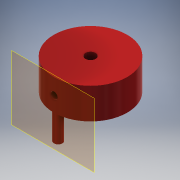
# Autodesk Inventor part: Cup_Dispenser_Transmission
Saved by Autodesk Inventor 2016 (Build 200138000, 138)
## iProperties
Created: 2015-07-09
Part Number: Cup_Dispenser_Transmission
Material: Generic
Document SubType Name: Modeling
Designer: 3DPrinterUser
Density: 1 g/cm^3
Appearance: Light Red
Author: 3DPrinterUser
Autodesk Inventor part; units mm, degrees
ref_plane "YZ Plane" through (0, 0, 0) normal (1, 0, 0) x (0, 1, 0)
ref_plane "XZ Plane" through (0, 0, 0) normal (0, 1, 0) x (-1, 0, 0)
ref_plane "XY Plane" through (0, 0, 0) normal (0, 0, 1) x (1, 0, 0)
sketch "Sketch1" plane through (0, 0, 0) normal (0, 0, 1) x (1, 0, 0)
  circle A0 centre (0, -63.4645) radius 57 construction
  circle A1 centre (0, -63.4645) radius 2.5 projected
  arc A2 (18.2706, -84.7351) -> (18.2706, -78.7351) centre (18.2706, -81.7351) ccw construction
  line L0 (18.2706, -78.7351) -> (-18.2706, -78.7351) construction
  line L1 (-18.2706, -84.7351) -> (18.2706, -84.7351) construction
  arc A3 (-18.2706, -78.7351) -> (-18.2706, -84.7351) centre (-18.2706, -81.7351) ccw construction
  line L2 (-18.2706, -81.7351) -> (18.2706, -81.7351) construction
  line L3 (0, -63.4645) -> (0, -81.7351) construction
  circle A4 centre (0, -81.7351) radius 3
  circle A5 centre (0, -63.4645) radius 21.2706
  point P0 (0, 0)
  point P1 (0, -84.7351)
  constraints: 4 end point, 2 coincident, 2 midpoint, 2 vertical alignment, 1 horizontal, 4 other
ref_plane "Work Plane1" through (-57, -120.4645, -15) normal (0, 0, -1) x (0, 1, 0)
extrude "Extrusion1" add sketch "Sketch1" against normal up to surface (15 mm away) contours A4
sketch "Sketch2" plane through (0, -81.7351, 0) normal (0, 0, 1) x (1, 0, 0)
  circle A0 centre (0, 18.2706) radius 21.2706 projected
  point P0 (0, 81.7351)
ref_plane "Work Plane2" through (-2, -65.4645, 3) normal (0, 0, -1) x (0, 1, 0)
extrude "Extrusion2" add sketch "Sketch2" along normal up to surface (3 mm away)
sketch "Sketch3" plane through (0, -63.4645, 3) normal (0, 0, 1) x (1, 0, 0)
  circle A0 centre (0, 0) radius 21.2706 projected
  circle A1 centre (0, 0) radius 2.5 projected
  point P0 (0, 63.4645)
  point P1 (0, -21.2706)
  constraints: 1 vertical alignment
extrude "Extrusion3" add sketch "Sketch3" along normal blind 15
ref_plane "Work Plane4" through (0, -84.7351, 0) normal (0, -1, 0) x (1, 0, 0)
ref_plane "Work Plane3" through (15.5, -84.4645, 27) normal (0, -1, 0) x (-1, 0, 0)
sketch "Sketch4" plane through (0, -84.7351, 0) normal (0, -1, 0) x (1, 0, 0)
  line L0 (21.2706, 18) -> (-21.2706, 18) construction
  line L1 (21.2706, 0) -> (-21.2706, 0) construction
  line L2 (0, 0) -> (0, 9) construction
  line L3 (0, 9) -> (0, 18) construction
  constraints: 4 end point, 1 coincident, 1 collinear, 1 midpoint, 1 vertical
hole "Hole1" at (0, -84.7351, 9) direction (0, 1, 0) diameter 4 end up to face face through (0, -63.4645, 3) facing (0, 0, 1) round with radius 2.5 far side yes
thicken "Thicken1" operation add thickness 0.6 both sides no extend neighbours yes toward (0, 0, 1) faces at (-0.4989, -54.4986, 0) (-7.669, -83.3045, 6) (-0.3679, -84.7125, -5) (0.5681, -80.4335, -15)
thicken "Thicken2" operation add thickness 0.4 both sides no extend neighbours yes toward (0.9967573, -0.0804666, 0) faces at (2.4919, -63.6657, 13)
equation "\"d4\" = 5 * thickness"
equation "\"thickness\" = 3"
body "Solid1"
